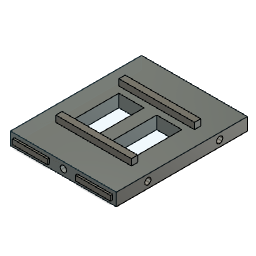
CircuitHolderBottomPlate (Autodesk Fusion 360 design; units mm, degrees)
Autodesk Fusion 360 part; units mm, degrees
sketch "Sketch1" plane through (0, 0, 0) normal (0, 1, 0) x (1, 0, 0)
  line L0 (0, 0) -> (42, 0)
  line L1 (0, 0) -> (-42, 0)
  line L2 (-42, 0) -> (-42, -104)
  line L3 (42, 0) -> (42, -104)
  line L4 (-42, -104) -> (42, -104)
  dimension "d1" = 42
  dimension "d2" = 42
  dimension "d3" = 104
  dimension "d4" = 104
  constraint coincident L0.start L1.start
  constraint horizontal L0
  constraint parallel L0 L1
  constraint perpendicular L1 L2
  constraint perpendicular L0 L3
  measures "d1" distance of L0.start L0.end
  measures "d2" distance of L0.start L1.end
  measures "d3" distance of L1.end L2.end
  measures "d4" distance of L0.end L3.end
extrude "Extrude1" add sketch "Sketch1" along normal blind 10
sketch "Sketch2" plane through (-42, 0, 0) normal (-1, 0, 0) x (0, 0, 1)
  line L0 (0, 0) -> (104, 0)
  line L1 (104, 0) -> (104, 10)
  line L2 (104, 10) -> (0, 10)
  line L3 (0, 10) -> (0, 0)
sketch "Sketch3" plane through (0, 0, 104) normal (0, 0, 1) x (1, 0, 0)
  line L0 (-42, 0) -> (42, 0)
  line L1 (42, 0) -> (42, 10)
  line L2 (42, 10) -> (-42, 10)
  line L3 (-42, 10) -> (-42, 0)
sketch "Sketch4" plane through (0, 0, 104) normal (0, 0, 1) x (1, 0, 0)
sketch "Sketch5" plane through (0, 0, 104) normal (0, 0, 1) x (1, 0, 0)
sketch "Sketch6" plane through (0, 0, 104) normal (0, 0, 1) x (1, 0, 0)
  line L0 (-39, 7) -> (-39, 3)
  line L1 (-39, 3) -> (-11, 3)
  line L2 (-11, 3) -> (-11, 7)
  line L3 (-11, 7) -> (-39, 7)
  dimension "d21" = 28
  constraint vertical L0
  constraint perpendicular L0 L1
  constraint perpendicular L1 L2
  constraint perpendicular L0 L3
  measures "d21" distance of L0.end L1.end
sketch "Sketch7" plane through (0, 0, 104) normal (0, 0, 1) x (1, 0, 0)
  line L0 (39, 5) -> (39, 3)
  line L1 (39, 3) -> (11, 3)
  line L2 (11, 3) -> (11, 7)
  line L3 (11, 7) -> (39, 7)
  line L4 (39, 7) -> (39, 5)
  circle A0 centre (0, 5) radius 2.5
  dimension "d22" = 28
  dimension "d23" = 5
  constraint perpendicular L0 L1
  constraint perpendicular L1 L2
  constraint perpendicular L2 L3
  measures "d22" distance of L0.end L1.end
  measures "d23" diameter of A0
extrude "Extrude2" add sketch "Sketch6" sketch "Sketch7" along normal blind 1.5 of sketch 2 contours L0 L1 L2 L3 L4
sketch "Sketch8" plane through (0, 0, 104) normal (0, 0, 1) x (1, 0, 0)
  circle A0 centre (0, 5) radius 2.5
  dimension "d26" = 5
  measures "d26" diameter of A0
extrude "Extrude3" cut sketch "Sketch8" against normal blind 25
sketch "Sketch9" plane through (0, 0, 0) normal (0, 0, -1) x (-1, 0, 0)
  line L0 (-42, 0) -> (42, 0)
  line L1 (42, 0) -> (42, 10)
  line L2 (42, 10) -> (-42, 10)
  line L3 (-42, 10) -> (-42, 0)
  circle A0 centre (0, 5) radius 2.5
  dimension "d29" = 5
  measures "d29" diameter of A0
extrude "Extrude4" cut sketch "Sketch9" against normal blind 25 contours A0
sketch "Sketch10" plane through (42, 0, 0) normal (1, 0, 0) x (0, 0, -1)
  line L0 (-104, 0) -> (0, 0)
  line L1 (0, 0) -> (0, 10)
  line L2 (0, 10) -> (-104, 10)
  line L3 (-104, 10) -> (-104, 0)
  circle A0 centre (-79, 5) radius 2.5
  circle A1 centre (-22, 5) radius 2.5
  dimension "d33" = 5
  dimension "d35" = 5
  measures "d33" diameter of A0
  measures "d35" diameter of A1
extrude "Extrude5" cut sketch "Sketch10" against normal blind 25 contours A0 | A1
sketch "Sketch11" plane through (-42, 0, 0) normal (-1, 0, 0) x (0, 0, 1)
  circle A0 centre (22, 5) radius 2.5
  circle A1 centre (82, 5) radius 2.5
  dimension "d39" = 5
  dimension "d41" = 5
  measures "d39" diameter of A0
  measures "d41" diameter of A1
extrude "Extrude6" cut sketch "Sketch11" against normal blind 25
sketch "Sketch12" plane through (0, 10, 0) normal (0, 1, 0) x (-1, 0, 0)
  line L0 (-42, 0) -> (42, 0)
  line L1 (42, 0) -> (42, 104)
  line L2 (42, 104) -> (-42, 104)
  line L3 (-42, 104) -> (-42, 0)
sketch "Sketch13" plane through (0, 10, 0) normal (0, 1, 0) x (-1, 0, 0)
  line L0 (-30, 80) -> (-30, 75)
  line L1 (-30, 75) -> (30, 75)
  line L2 (30, 75) -> (30, 80)
  line L3 (30, 80) -> (-30, 80)
  line L4 (-30, 30) -> (30, 30)
  line L5 (30, 30) -> (30, 25)
  line L6 (30, 25) -> (-30, 25)
  line L7 (-30, 25) -> (-30, 30)
  dimension "d44" = 5
  dimension "d45" = 5
  constraint vertical L0
  constraint perpendicular L0 L1
  constraint perpendicular L1 L2
  constraint perpendicular L0 L3
  constraint perpendicular L0 L4
  constraint perpendicular L4 L5
  constraint perpendicular L5 L6
  constraint perpendicular L4 L7
  measures "d44" distance of L0.start L0.end
  measures "d45" distance of L4.end L5.end
extrude "Extrude7" add sketch "Sketch13" along normal blind 5
sketch "Sketch14" plane through (0, 10, 0) normal (0, 1, 0) x (-1, 0, 0)
  line L0 (25, 35) -> (5, 35)
  line L1 (5, 35) -> (5, 70)
  line L2 (5, 70) -> (25, 70)
  line L3 (25, 70) -> (25, 35)
  line L4 (-5, 35) -> (-25, 35)
  line L5 (-25, 35) -> (-25, 70)
  line L6 (-25, 70) -> (-5, 70)
  line L7 (-5, 70) -> (-5, 35)
  constraint horizontal L0
  constraint perpendicular L0 L1
  constraint perpendicular L1 L2
  constraint perpendicular L0 L3
  constraint perpendicular L3 L4
  constraint perpendicular L4 L5
  constraint perpendicular L3 L6
  constraint perpendicular L4 L7
extrude "Extrude8" cut sketch "Sketch14" against normal blind 20
